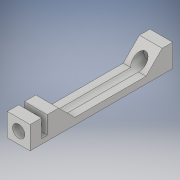
# Autodesk Inventor part: ptfe_cutter_v6_40mm
Saved by Autodesk Inventor 2019.4 (Build 234330000, 330)
## iProperties
Created: 2020-10-22
Part Number: ptfe_cutter_v6_40mm
Material: Generic
Document SubType Name: Modeling
Designer: PSHUGHAM
Density: 1 g/cm^3
Appearance: Default
Author: PSHUGHAM
Autodesk Inventor part; units mm, degrees
ref_plane "YZ Plane" through (0, 0, 0) normal (1, 0, 0) x (0, 1, 0)
ref_plane "XZ Plane" through (0, 0, 0) normal (0, 1, 0) x (-1, 0, 0)
ref_plane "XY Plane" through (0, 0, 0) normal (0, 0, 1) x (1, 0, 0)
sketch "Sketch1" plane through (0, 0, 0) normal (0, 1, 0) x (-1, 0, 0)
  line L0 (0, 0) -> (8, 0)
  line L1 (8, 0) -> (8, -50)
  line L2 (8, -50) -> (0, -50)
  line L3 (0, -50) -> (0, 0)
  dimension "d0" = 8
  dimension "d1" = 50
  constraints: 8 end point, 2 parallel, 1 horizontal, 1 perpendicular
  measures "d0" distance of L1.end L2.end
  measures "d1" distance of L0.end L1.end
extrude "Extrusion1" add sketch "Sketch1" along normal blind 8
sketch "Sketch2" plane through (-8, 0, 0) normal (0, 0, 1) x (1, 0, 0)
  circle A0 centre (4, 4) radius 2.15
  point P0 (8, 0)
  dimension "d4" = 4.3
  constraints: 1 centre point
  measures "d4" diameter of A0
extrude "Extrusion2" cut sketch "Sketch2" against normal blind 4
sketch "Sketch3" plane through (0, 8, 0) normal (0, 1, 0) x (1, 0, 0)
  line L0 (-10.8104, 6) -> (3.7678, 6)
  line L1 (3.7678, 6) -> (3.7678, 4)
  line L2 (3.7678, 4) -> (-10.8104, 4)
  line L3 (-10.8104, 4) -> (-10.8104, 6)
  line L4 (-8, 0) -> (0, 0) projected
  dimension "d8" = 2
  dimension "d9" = 4
  constraints: 8 end point, 2 parallel, 1 horizontal, 1 perpendicular
  measures "d8" distance of L2.end L0.start
  measures "d9" distance between parallel lines of L2 L4
extrude "Extrusion3" cut sketch "Sketch3" against normal blind 6.2
sketch "Sketch4" plane through (-8, 8, -6) normal (0, 0, 1) x (1, 0, 0)
  circle A0 centre (4, -4) radius 2.15 projected
  circle A1 centre (4, -4) radius 2.15
  point P0 (8, -8)
  constraints: 1 centre point, 1 coincident
extrude "Extrusion4" cut sketch "Sketch4" against normal blind 40
sketch "Sketch5" plane through (0, 0, 0) normal (1, 0, 0) x (0, 0, -1)
  line L0 (6, 8) -> (50, 8) projected
  line L1 (6, 8) -> (10, 8)
  line L2 (10, 8) -> (15.6569, 2.3431)
  line L3 (15.6569, 2.3431) -> (40.6569, 2.3431)
  line L4 (6, 1.85) -> (46, 1.85) projected
  line L5 (40.6569, 2.3431) -> (46.3137, 8)
  line L6 (46.3137, 8) -> (10, 8)
  point P0 (0, 0)
  dimension "d14" = 4
  dimension "d15" = 8
  dimension "d16" = 135
  dimension "d17" = 25
  dimension "d18" = 135
  constraints: 10 end point, 2 point on line, 1 collinear, 1 parallel, 1 perpendicular
  measures "d14" distance of L0.start L1.end
  measures "d15" distance of L1.end L2.end
  measures "d16" angle of L1 L2
  measures "d17" distance of L2.end L3.end
  measures "d18" angle of L3 L2
extrude "Extrusion5" cut sketch "Sketch5" against normal blind 40
body "Solid1"
